Autodesk Fusion 360 part; units mm, degrees
(part 2 of 5)
sketch "草图10 (3)" plane through (0, 0, 26) normal (0, 0, 1) x (1, 0, 0) in component "L2_RemovableGrate"
  line L0 (329, 60.3) -> (333, 60.3)
  line L1 (333, 60.3) -> (333, 129.7)
  line L2 (333, 129.7) -> (329, 129.7)
  line L3 (329, 129.7) -> (329, 60.3)
  dimension "d585" = 329
  dimension "d587" = 4
  dimension "d588" = 69.4
  constraint horizontal L0
  constraint vertical L1
  constraint horizontal L2
  constraint vertical L3
  measures "d585" horizontal distance of origin L0.start
  measures "d587" horizontal distance of L0.start L0.end
  measures "d588" vertical distance of L0.end L1.end
extrude "Drain slot 9''" cut sketch "草图10 (3)" along normal blind 4 bodies 6 in component "L2_RemovableGrate"
ref_plane "工作平面11" through (0, 0, 26) normal (0, 0, 1) x (1, 0, 0) in component "L2_RemovableGrate"
sketch "草图11 (3)" plane through (0, 0, 26) normal (0, 0, 1) x (1, 0, 0) in component "L2_RemovableGrate"
  line L0 (339, 60.3) -> (343, 60.3)
  line L1 (343, 60.3) -> (343, 129.7)
  line L2 (343, 129.7) -> (339, 129.7)
  line L3 (339, 129.7) -> (339, 60.3)
  dimension "d593" = 339
  dimension "d595" = 4
  dimension "d596" = 69.4
  constraint horizontal L0
  constraint vertical L1
  constraint horizontal L2
  constraint vertical L3
  measures "d593" horizontal distance of origin L0.start
  measures "d595" horizontal distance of L0.start L0.end
  measures "d596" vertical distance of L0.end L1.end
extrude "Drain slot 10''" cut sketch "草图11 (3)" along normal blind 4 bodies 6 in component "L2_RemovableGrate"
ref_plane "工作平面12" through (0, 0, 26) normal (0, 0, 1) x (1, 0, 0) in component "L2_RemovableGrate"
sketch "草图12 (3)" plane through (0, 0, 26) normal (0, 0, 1) x (1, 0, 0) in component "L2_RemovableGrate"
  line L0 (349, 60.3) -> (353, 60.3)
  line L1 (353, 60.3) -> (353, 129.7)
  line L2 (353, 129.7) -> (349, 129.7)
  line L3 (349, 129.7) -> (349, 60.3)
  dimension "d601" = 349
  dimension "d603" = 4
  dimension "d604" = 69.4
  constraint horizontal L0
  constraint vertical L1
  constraint horizontal L2
  constraint vertical L3
  measures "d601" horizontal distance of origin L0.start
  measures "d603" horizontal distance of L0.start L0.end
  measures "d604" vertical distance of L0.end L1.end
extrude "Drain slot 11''" cut sketch "草图12 (3)" along normal blind 4 bodies 6 in component "L2_RemovableGrate"
ref_plane "工作平面13" through (0, 0, 26) normal (0, 0, 1) x (1, 0, 0) in component "L2_RemovableGrate"
sketch "草图13 (2)" plane through (0, 0, 26) normal (0, 0, 1) x (1, 0, 0) in component "L2_RemovableGrate"
  line L0 (359, 60.3) -> (363, 60.3)
  line L1 (363, 60.3) -> (363, 129.7)
  line L2 (363, 129.7) -> (359, 129.7)
  line L3 (359, 129.7) -> (359, 60.3)
  dimension "d609" = 359
  dimension "d611" = 4
  dimension "d612" = 69.4
  constraint horizontal L0
  constraint vertical L1
  constraint horizontal L2
  constraint vertical L3
  measures "d609" horizontal distance of origin L0.start
  measures "d611" horizontal distance of L0.start L0.end
  measures "d612" vertical distance of L0.end L1.end
extrude "Drain slot 12'" cut sketch "草图13 (2)" along normal blind 4 bodies 6 in component "L2_RemovableGrate"
ref_plane "工作平面14" through (0, 0, 26) normal (0, 0, 1) x (1, 0, 0) in component "L2_RemovableGrate"
sketch "草图14 (2)" plane through (0, 0, 26) normal (0, 0, 1) x (1, 0, 0) in component "L2_RemovableGrate"
  line L0 (369, 60.3) -> (373, 60.3)
  line L1 (373, 60.3) -> (373, 129.7)
  line L2 (373, 129.7) -> (369, 129.7)
  line L3 (369, 129.7) -> (369, 60.3)
  dimension "d617" = 369
  dimension "d619" = 4
  dimension "d620" = 69.4
  constraint horizontal L0
  constraint vertical L1
  constraint horizontal L2
  constraint vertical L3
  measures "d617" horizontal distance of origin L0.start
  measures "d619" horizontal distance of L0.start L0.end
  measures "d620" vertical distance of L0.end L1.end
extrude "Drain slot 13'" cut sketch "草图14 (2)" along normal blind 4 bodies 6 in component "L2_RemovableGrate"
ref_plane "工作平面15" through (0, 0, 26) normal (0, 0, 1) x (1, 0, 0) in component "L2_RemovableGrate"
sketch "草图15 (2)" plane through (0, 0, 26) normal (0, 0, 1) x (1, 0, 0) in component "L2_RemovableGrate"
  line L0 (379, 60.3) -> (383, 60.3)
  line L1 (383, 60.3) -> (383, 129.7)
  line L2 (383, 129.7) -> (379, 129.7)
  line L3 (379, 129.7) -> (379, 60.3)
  dimension "d625" = 379
  dimension "d627" = 4
  dimension "d628" = 69.4
  constraint horizontal L0
  constraint vertical L1
  constraint horizontal L2
  constraint vertical L3
  measures "d625" horizontal distance of origin L0.start
  measures "d627" horizontal distance of L0.start L0.end
  measures "d628" vertical distance of L0.end L1.end
extrude "Drain slot 14'" cut sketch "草图15 (2)" along normal blind 4 bodies 6 in component "L2_RemovableGrate"
ref_plane "工作平面16" through (0, 0, 26) normal (0, 0, 1) x (1, 0, 0) in component "L2_RemovableGrate"
sketch "草图16 (2)" plane through (0, 0, 26) normal (0, 0, 1) x (1, 0, 0) in component "L2_RemovableGrate"
  line L0 (389, 60.3) -> (393, 60.3)
  line L1 (393, 60.3) -> (393, 129.7)
  line L2 (393, 129.7) -> (389, 129.7)
  line L3 (389, 129.7) -> (389, 60.3)
  dimension "d633" = 389
  dimension "d635" = 4
  dimension "d636" = 69.4
  constraint horizontal L0
  constraint vertical L1
  constraint horizontal L2
  constraint vertical L3
  measures "d633" horizontal distance of origin L0.start
  measures "d635" horizontal distance of L0.start L0.end
  measures "d636" vertical distance of L0.end L1.end
extrude "Drain slot 15'" cut sketch "草图16 (2)" along normal blind 4 bodies 6 in component "L2_RemovableGrate"
ref_plane "工作平面17" through (0, 0, 26) normal (0, 0, 1) x (1, 0, 0) in component "L2_RemovableGrate"
sketch "草图17" plane through (0, 0, 26) normal (0, 0, 1) x (1, 0, 0) in component "L2_RemovableGrate"
  line L0 (399, 60.3) -> (403, 60.3)
  line L1 (403, 60.3) -> (403, 129.7)
  line L2 (403, 129.7) -> (399, 129.7)
  line L3 (399, 129.7) -> (399, 60.3)
  dimension "d641" = 399
  dimension "d643" = 4
  dimension "d644" = 69.4
  constraint horizontal L0
  constraint vertical L1
  constraint horizontal L2
  constraint vertical L3
  measures "d641" horizontal distance of origin L0.start
  measures "d643" horizontal distance of L0.start L0.end
  measures "d644" vertical distance of L0.end L1.end
extrude "Drain slot 16" cut sketch "草图17" along normal blind 4 bodies 6 in component "L2_RemovableGrate"
ref_plane "工作平面18" through (0, 0, 26) normal (0, 0, 1) x (1, 0, 0) in component "L2_RemovableGrate"
sketch "草图18" plane through (0, 0, 26) normal (0, 0, 1) x (1, 0, 0) in component "L2_RemovableGrate"
  line L0 (409, 60.3) -> (413, 60.3)
  line L1 (413, 60.3) -> (413, 129.7)
  line L2 (413, 129.7) -> (409, 129.7)
  line L3 (409, 129.7) -> (409, 60.3)
  dimension "d649" = 409
  dimension "d651" = 4
  dimension "d652" = 69.4
  constraint horizontal L0
  constraint vertical L1
  constraint horizontal L2
  constraint vertical L3
  measures "d649" horizontal distance of origin L0.start
  measures "d651" horizontal distance of L0.start L0.end
  measures "d652" vertical distance of L0.end L1.end
extrude "Drain slot 17" cut sketch "草图18" along normal blind 4 bodies 6 in component "L2_RemovableGrate"
chamfer "倒角1'''''" distance 0.4 angle 45 4 edges at (331, 136.7, 30) (426.7, 95, 30) (331, 53.3, 30) (235.3, 95, 30) on bodies 6 in component "L2_RemovableGrate"
ref_plane "工作平面1" through (0, 0, 10) normal (0, 0, 1) x (1, 0, 0) in component "R2_Integrated"
sketch "草图1 (7)" plane through (0, 0, 10) normal (0, 0, 1) x (1, 0, 0) in component "R2_Integrated"
  line L0 (726, 50) -> (860, 50)
  line L1 (860, 50) -> (860, 140)
  line L2 (860, 140) -> (726, 140)
  line L3 (726, 140) -> (726, 50)
  dimension "d658" = 726
  dimension "d659" = 50
  dimension "d660" = 134
  dimension "d661" = 90
  constraint horizontal L0
  constraint vertical L1
  constraint horizontal L2
  constraint vertical L3
  measures "d658" horizontal distance of origin L0.start
  measures "d659" vertical distance of origin L0.start
  measures "d660" horizontal distance of L0.start L0.end
  measures "d661" vertical distance of L0.end L1.end
extrude "R05 pan blank'''" add sketch "草图1 (7)" along normal blind 25 separate body makes body 7 in component "R2_Integrated"
fillet "Outside corner rounds'''" radius 3 4 edges at (726, 140, 22.5) (860, 140, 22.5) (860, 50, 22.5) (726, 50, 22.5) on bodies 7 in component "R2_Integrated"
ref_plane "工作平面2" through (729, 0, 0) normal (1, 0, 0) x (0, 1, 0) in component "R2_Integrated"
sketch "草图2 (7)" plane through (729, 0, 0) normal (1, 0, 0) x (0, 0, -1) in component "R2_Integrated"
  line L0 (-22.1441, 53) -> (-13, 140)
  line L1 (-13, 140) -> (-36, 140)
  line L2 (-36, 140) -> (-36, 53)
  line L3 (-36, 53) -> (-22.1441, 53)
  dimension "d670" = 13
  dimension "d672" = 36
  constraint horizontal L1
  constraint vertical L2
  constraint horizontal L3
  measures "d670" horizontal distance of origin L0.end
  measures "d672" horizontal distance of origin L1.end
extrude "R05 continuous slope and open edge'''" cut sketch "草图2 (7)" along normal blind 128 bodies 7 in component "R2_Integrated"
ref_plane "工作平面3" through (0, 0, 10) normal (0, 0, 1) x (1, 0, 0) in component "R2_Integrated"
sketch "草图3 (7)" plane through (0, 0, 10) normal (0, 0, 1) x (1, 0, 0) in component "R2_Integrated"
  line L0 (729, 53) -> (736, 65)
  line L1 (736, 65) -> (729, 77)
  line L2 (729, 77) -> (729, 53)
  dimension "d677" = 729
  dimension "d679" = 736
  dimension "d680" = 65
  constraint vertical L2
  measures "d677" horizontal distance of origin L0.start
  measures "d679" horizontal distance of origin L0.end
  measures "d680" vertical distance of origin L0.end
extrude "R05 triangular flow seat 00'''" add sketch "草图3 (7)" along normal blind 16 bodies 7 in component "R2_Integrated"
fillet "R05 soften flow seat tip'''" radius 1 1 edges at (736, 65, 23.4414) on bodies 7 in component "R2_Integrated"
ref_plane "工作平面4" through (0, 0, 10) normal (0, 0, 1) x (1, 0, 0) in component "R2_Integrated"
sketch "草图4 (7)" plane through (0, 0, 10) normal (0, 0, 1) x (1, 0, 0) in component "R2_Integrated"
  line L0 (729, 113) -> (736, 125)
  line L1 (736, 125) -> (729, 137)
  line L2 (729, 137) -> (729, 113)
  dimension "d688" = 729
  dimension "d690" = 736
  dimension "d691" = 125
  constraint vertical L2
  measures "d688" horizontal distance of origin L0.start
  measures "d690" horizontal distance of origin L0.end
  measures "d691" vertical distance of origin L0.end
extrude "R05 triangular flow seat 01'''" add sketch "草图4 (7)" along normal blind 16 bodies 7 in component "R2_Integrated"
fillet "R05 soften flow seat tip (1)'''" radius 1 1 edges at (736, 125, 20.2883) on bodies 7 in component "R2_Integrated"
ref_plane "工作平面5" through (0, 0, 10) normal (0, 0, 1) x (1, 0, 0) in component "R2_Integrated"
sketch "草图5 (7)" plane through (0, 0, 10) normal (0, 0, 1) x (1, 0, 0) in component "R2_Integrated"
  line L0 (857, 53) -> (850, 65)
  line L1 (850, 65) -> (857, 77)
  line L2 (857, 77) -> (857, 53)
  dimension "d699" = 857
  dimension "d701" = 850
  dimension "d702" = 65
  constraint vertical L2
  measures "d699" horizontal distance of origin L0.start
  measures "d701" horizontal distance of origin L0.end
  measures "d702" vertical distance of origin L0.end
extrude "R05 triangular flow seat 10'''" add sketch "草图5 (7)" along normal blind 16 bodies 7 in component "R2_Integrated"
fillet "R05 soften flow seat tip (2)'''" radius 1 1 edges at (850, 65, 23.4414) on bodies 7 in component "R2_Integrated"
ref_plane "工作平面6" through (0, 0, 10) normal (0, 0, 1) x (1, 0, 0) in component "R2_Integrated"
sketch "草图6 (7)" plane through (0, 0, 10) normal (0, 0, 1) x (1, 0, 0) in component "R2_Integrated"
  line L0 (857, 113) -> (850, 125)
  line L1 (850, 125) -> (857, 137)
  line L2 (857, 137) -> (857, 113)
  dimension "d710" = 857
  dimension "d712" = 850
  dimension "d713" = 125
  constraint vertical L2
  measures "d710" horizontal distance of origin L0.start
  measures "d712" horizontal distance of origin L0.end
  measures "d713" vertical distance of origin L0.end
extrude "R05 triangular flow seat 11'''" add sketch "草图6 (7)" along normal blind 16 bodies 7 in component "R2_Integrated"
fillet "R05 soften flow seat tip (3)'''" radius 1 1 edges at (850, 125, 20.2883) on bodies 7 in component "R2_Integrated"
ref_plane "工作平面7" through (0, 0, 0) normal (0, 0, 1) x (1, 0, 0) in component "R2_Integrated"
sketch "草图7 (7)" plane through (0, 0, 0) normal (0, 0, 1) x (1, 0, 0) in component "R2_Integrated"
  line L0 (729, 50) -> (737, 50)
  line L1 (737, 50) -> (737, 131)
  line L2 (737, 131) -> (729, 131)
  line L3 (729, 131) -> (729, 50)
  dimension "d721" = 729
  dimension "d722" = 50
  dimension "d723" = 8
  dimension "d724" = 81
  constraint horizontal L0
  constraint vertical L1
  constraint horizontal L2
  constraint vertical L3
  measures "d721" horizontal distance of origin L0.start
  measures "d722" vertical distance of origin L0.start
  measures "d723" horizontal distance of L0.start L0.end
  measures "d724" vertical distance of L0.end L1.end
extrude "R05 low integral runner 0'''" add sketch "草图7 (7)" along normal blind 10 bodies 7 in component "R2_Integrated"
ref_plane "工作平面8" through (0, 0, 0) normal (0, 0, 1) x (1, 0, 0) in component "R2_Integrated"
sketch "草图8 (7)" plane through (0, 0, 0) normal (0, 0, 1) x (1, 0, 0) in component "R2_Integrated"
  line L0 (849, 50) -> (857, 50)
  line L1 (857, 50) -> (857, 131)
  line L2 (857, 131) -> (849, 131)
  line L3 (849, 131) -> (849, 50)
  dimension "d729" = 849
  dimension "d730" = 50
  dimension "d731" = 8
  dimension "d732" = 81
  constraint horizontal L0
  constraint vertical L1
  constraint horizontal L2
  constraint vertical L3
  measures "d729" horizontal distance of origin L0.start
  measures "d730" vertical distance of origin L0.start
  measures "d731" horizontal distance of L0.start L0.end
  measures "d732" vertical distance of L0.end L1.end
extrude "R05 low integral runner 1'''" add sketch "草图8 (7)" along normal blind 10 bodies 7 in component "R2_Integrated"
chamfer "倒角1''''''" distance 0.4 angle 45 5 edges at (729, 96.5, 35) (857, 96.5, 35) (793, 53, 35) (726, 95, 35) (860, 95, 35) on bodies 7 in component "R2_Integrated"
ref_plane "工作平面1" through (0, 0, 26) normal (0, 0, 1) x (1, 0, 0) in component "R2_RemovableGrate"
sketch "草图1 (8)" plane through (0, 0, 26) normal (0, 0, 1) x (1, 0, 0) in component "R2_RemovableGrate"
  line L0 (729.3, 53.3) -> (856.7, 53.3)
  line L1 (856.7, 53.3) -> (856.7, 136.7)
  line L2 (856.7, 136.7) -> (729.3, 136.7)
  line L3 (729.3, 136.7) -> (729.3, 53.3)
  dimension "d738" = 729.3
  dimension "d740" = 127.4
  dimension "d741" = 83.4
  constraint horizontal L0
  constraint vertical L1
  constraint horizontal L2
  constraint vertical L3
  measures "d738" horizontal distance of origin L0.start
  measures "d740" horizontal distance of L0.start L0.end
  measures "d741" vertical distance of L0.end L1.end
extrude "Horizontal removable deck'''" add sketch "草图1 (8)" along normal blind 4 separate body makes body 8 in component "R2_RemovableGrate"
ref_plane "工作平面2" through (0, 0, 26) normal (0, 0, 1) x (1, 0, 0) in component "R2_RemovableGrate"
sketch "草图2 (8)" plane through (0, 0, 26) normal (0, 0, 1) x (1, 0, 0) in component "R2_RemovableGrate"
  line L0 (741, 60.3) -> (745, 60.3)
  line L1 (745, 60.3) -> (745, 129.7)
  line L2 (745, 129.7) -> (741, 129.7)
  line L3 (741, 129.7) -> (741, 60.3)
  dimension "d746" = 741
  dimension "d748" = 4
  dimension "d749" = 69.4
  constraint horizontal L0
  constraint vertical L1
  constraint horizontal L2
  constraint vertical L3
  measures "d746" horizontal distance of origin L0.start
  measures "d748" horizontal distance of L0.start L0.end
  measures "d749" vertical distance of L0.end L1.end
extrude "Drain slot 1'''" cut sketch "草图2 (8)" along normal blind 4 bodies 8 in component "R2_RemovableGrate"
ref_plane "工作平面3" through (0, 0, 26) normal (0, 0, 1) x (1, 0, 0) in component "R2_RemovableGrate"
sketch "草图3 (8)" plane through (0, 0, 26) normal (0, 0, 1) x (1, 0, 0) in component "R2_RemovableGrate"
  line L0 (751, 60.3) -> (755, 60.3)
  line L1 (755, 60.3) -> (755, 129.7)
  line L2 (755, 129.7) -> (751, 129.7)
  line L3 (751, 129.7) -> (751, 60.3)
  dimension "d754" = 751
  dimension "d756" = 4
  dimension "d757" = 69.4
  constraint horizontal L0
  constraint vertical L1
  constraint horizontal L2
  constraint vertical L3
  measures "d754" horizontal distance of origin L0.start
  measures "d756" horizontal distance of L0.start L0.end
  measures "d757" vertical distance of L0.end L1.end
extrude "Drain slot 2'''" cut sketch "草图3 (8)" along normal blind 4 bodies 8 in component "R2_RemovableGrate"
ref_plane "工作平面4" through (0, 0, 26) normal (0, 0, 1) x (1, 0, 0) in component "R2_RemovableGrate"
sketch "草图4 (8)" plane through (0, 0, 26) normal (0, 0, 1) x (1, 0, 0) in component "R2_RemovableGrate"
  line L0 (761, 60.3) -> (765, 60.3)
  line L1 (765, 60.3) -> (765, 129.7)
  line L2 (765, 129.7) -> (761, 129.7)
  line L3 (761, 129.7) -> (761, 60.3)
  dimension "d762" = 761
  dimension "d764" = 4
  dimension "d765" = 69.4
  constraint horizontal L0
  constraint vertical L1
  constraint horizontal L2
  constraint vertical L3
  measures "d762" horizontal distance of origin L0.start
  measures "d764" horizontal distance of L0.start L0.end
  measures "d765" vertical distance of L0.end L1.end
extrude "Drain slot 3'''" cut sketch "草图4 (8)" along normal blind 4 bodies 8 in component "R2_RemovableGrate"
ref_plane "工作平面5" through (0, 0, 26) normal (0, 0, 1) x (1, 0, 0) in component "R2_RemovableGrate"
sketch "草图5 (8)" plane through (0, 0, 26) normal (0, 0, 1) x (1, 0, 0) in component "R2_RemovableGrate"
  line L0 (771, 60.3) -> (775, 60.3)
  line L1 (775, 60.3) -> (775, 129.7)
  line L2 (775, 129.7) -> (771, 129.7)
  line L3 (771, 129.7) -> (771, 60.3)
  dimension "d770" = 771
  dimension "d772" = 4
  dimension "d773" = 69.4
  constraint horizontal L0
  constraint vertical L1
  constraint horizontal L2
  constraint vertical L3
  measures "d770" horizontal distance of origin L0.start
  measures "d772" horizontal distance of L0.start L0.end
  measures "d773" vertical distance of L0.end L1.end
extrude "Drain slot 4'''" cut sketch "草图5 (8)" along normal blind 4 bodies 8 in component "R2_RemovableGrate"
ref_plane "工作平面6" through (0, 0, 26) normal (0, 0, 1) x (1, 0, 0) in component "R2_RemovableGrate"
sketch "草图6 (8)" plane through (0, 0, 26) normal (0, 0, 1) x (1, 0, 0) in component "R2_RemovableGrate"
  line L0 (781, 60.3) -> (785, 60.3)
  line L1 (785, 60.3) -> (785, 129.7)
  line L2 (785, 129.7) -> (781, 129.7)
  line L3 (781, 129.7) -> (781, 60.3)
  dimension "d778" = 781
  dimension "d780" = 4
  dimension "d781" = 69.4
  constraint horizontal L0
  constraint vertical L1
  constraint horizontal L2
  constraint vertical L3
  measures "d778" horizontal distance of origin L0.start
  measures "d780" horizontal distance of L0.start L0.end
  measures "d781" vertical distance of L0.end L1.end
extrude "Drain slot 5'''" cut sketch "草图6 (8)" along normal blind 4 bodies 8 in component "R2_RemovableGrate"
ref_plane "工作平面7" through (0, 0, 26) normal (0, 0, 1) x (1, 0, 0) in component "R2_RemovableGrate"
sketch "草图7 (8)" plane through (0, 0, 26) normal (0, 0, 1) x (1, 0, 0) in component "R2_RemovableGrate"
  line L0 (791, 60.3) -> (795, 60.3)
  line L1 (795, 60.3) -> (795, 129.7)
  line L2 (795, 129.7) -> (791, 129.7)
  line L3 (791, 129.7) -> (791, 60.3)
  dimension "d786" = 791
  dimension "d788" = 4
  dimension "d789" = 69.4
  constraint horizontal L0
  constraint vertical L1
  constraint horizontal L2
  constraint vertical L3
  measures "d786" horizontal distance of origin L0.start
  measures "d788" horizontal distance of L0.start L0.end
  measures "d789" vertical distance of L0.end L1.end
extrude "Drain slot 6'''" cut sketch "草图7 (8)" along normal blind 4 bodies 8 in component "R2_RemovableGrate"
ref_plane "工作平面8" through (0, 0, 26) normal (0, 0, 1) x (1, 0, 0) in component "R2_RemovableGrate"
sketch "草图8 (8)" plane through (0, 0, 26) normal (0, 0, 1) x (1, 0, 0) in component "R2_RemovableGrate"
  line L0 (801, 60.3) -> (805, 60.3)
  line L1 (805, 60.3) -> (805, 129.7)
  line L2 (805, 129.7) -> (801, 129.7)
  line L3 (801, 129.7) -> (801, 60.3)
  dimension "d794" = 801
  dimension "d796" = 4
  dimension "d797" = 69.4
  constraint horizontal L0
  constraint vertical L1
  constraint horizontal L2
  constraint vertical L3
  measures "d794" horizontal distance of origin L0.start
  measures "d796" horizontal distance of L0.start L0.end
  measures "d797" vertical distance of L0.end L1.end
extrude "Drain slot 7'''" cut sketch "草图8 (8)" along normal blind 4 bodies 8 in component "R2_RemovableGrate"
ref_plane "工作平面9" through (0, 0, 26) normal (0, 0, 1) x (1, 0, 0) in component "R2_RemovableGrate"
sketch "草图9 (4)" plane through (0, 0, 26) normal (0, 0, 1) x (1, 0, 0) in component "R2_RemovableGrate"
  line L0 (811, 60.3) -> (815, 60.3)
  line L1 (815, 60.3) -> (815, 129.7)
  line L2 (815, 129.7) -> (811, 129.7)
  line L3 (811, 129.7) -> (811, 60.3)
  dimension "d802" = 811
  dimension "d804" = 4
  dimension "d805" = 69.4
  constraint horizontal L0
  constraint vertical L1
  constraint horizontal L2
  constraint vertical L3
  measures "d802" horizontal distance of origin L0.start
  measures "d804" horizontal distance of L0.start L0.end
  measures "d805" vertical distance of L0.end L1.end
extrude "Drain slot 8'''" cut sketch "草图9 (4)" along normal blind 4 bodies 8 in component "R2_RemovableGrate"
ref_plane "工作平面10" through (0, 0, 26) normal (0, 0, 1) x (1, 0, 0) in component "R2_RemovableGrate"
sketch "草图10 (4)" plane through (0, 0, 26) normal (0, 0, 1) x (1, 0, 0) in component "R2_RemovableGrate"
  line L0 (821, 60.3) -> (825, 60.3)
  line L1 (825, 60.3) -> (825, 129.7)
  line L2 (825, 129.7) -> (821, 129.7)
  line L3 (821, 129.7) -> (821, 60.3)
  dimension "d810" = 821
  dimension "d812" = 4
  dimension "d813" = 69.4
  constraint horizontal L0
  constraint vertical L1
  constraint horizontal L2
  constraint vertical L3
  measures "d810" horizontal distance of origin L0.start
  measures "d812" horizontal distance of L0.start L0.end
  measures "d813" vertical distance of L0.end L1.end
extrude "Drain slot 9'''" cut sketch "草图10 (4)" along normal blind 4 bodies 8 in component "R2_RemovableGrate"
ref_plane "工作平面11" through (0, 0, 26) normal (0, 0, 1) x (1, 0, 0) in component "R2_RemovableGrate"
sketch "草图11 (4)" plane through (0, 0, 26) normal (0, 0, 1) x (1, 0, 0) in component "R2_RemovableGrate"
  line L0 (831, 60.3) -> (835, 60.3)
  line L1 (835, 60.3) -> (835, 129.7)
  line L2 (835, 129.7) -> (831, 129.7)
  line L3 (831, 129.7) -> (831, 60.3)
  dimension "d818" = 831
  dimension "d820" = 4
  dimension "d821" = 69.4
  constraint horizontal L0
  constraint vertical L1
  constraint horizontal L2
  constraint vertical L3
  measures "d818" horizontal distance of origin L0.start
  measures "d820" horizontal distance of L0.start L0.end
  measures "d821" vertical distance of L0.end L1.end
extrude "Drain slot 10'''" cut sketch "草图11 (4)" along normal blind 4 bodies 8 in component "R2_RemovableGrate"
ref_plane "工作平面12" through (0, 0, 26) normal (0, 0, 1) x (1, 0, 0) in component "R2_RemovableGrate"
sketch "草图12 (4)" plane through (0, 0, 26) normal (0, 0, 1) x (1, 0, 0) in component "R2_RemovableGrate"
  line L0 (841, 60.3) -> (845, 60.3)
  line L1 (845, 60.3) -> (845, 129.7)
  line L2 (845, 129.7) -> (841, 129.7)
  line L3 (841, 129.7) -> (841, 60.3)
  dimension "d826" = 841
  dimension "d828" = 4
  dimension "d829" = 69.4
  constraint horizontal L0
  constraint vertical L1
  constraint horizontal L2
  constraint vertical L3
  measures "d826" horizontal distance of origin L0.start
  measures "d828" horizontal distance of L0.start L0.end
  measures "d829" vertical distance of L0.end L1.end
extrude "Drain slot 11'''" cut sketch "草图12 (4)" along normal blind 4 bodies 8 in component "R2_RemovableGrate"
chamfer "倒角1'''''''" distance 0.4 angle 45 4 edges at (793, 136.7, 30) (856.7, 95, 30) (793, 53.3, 30) (729.3, 95, 30) on bodies 8 in component "R2_RemovableGrate"
ref_plane "工作平面1" through (0, 0, 10) normal (0, 0, 1) x (1, 0, 0) in component "LS_Integrated"
sketch "草图1 (9)" plane through (0, 0, 10) normal (0, 0, 1) x (1, 0, 0) in component "LS_Integrated"
  line L0 (50, 142) -> (170, 142)
  line L1 (170, 142) -> (170, 322)
  line L2 (170, 322) -> (50, 322)
  line L3 (50, 322) -> (50, 142)
  dimension "d835" = 50
  dimension "d836" = 142
  dimension "d837" = 120
  dimension "d838" = 180
  constraint horizontal L0
  constraint vertical L1
  constraint horizontal L2
  constraint vertical L3
  measures "d835" horizontal distance of origin L0.start
  measures "d836" vertical distance of origin L0.start
  measures "d837" horizontal distance of L0.start L0.end
  measures "d838" vertical distance of L0.end L1.end
extrude "R05 pan blank''''" add sketch "草图1 (9)" along normal blind 25 separate body makes body 9 in component "LS_Integrated"
fillet "Outside corner rounds''''" radius 3 4 edges at (50, 322, 22.5) (170, 322, 22.5) (170, 142, 22.5) (50, 142, 22.5) on bodies 9 in component "LS_Integrated"
ref_plane "工作平面2" through (0, 319, 0) normal (0, 1, 0) x (0, 0, 1) in component "LS_Integrated"
sketch "草图2 (9)" plane through (0, 319, 0) normal (0, 1, 0) x (1, 0, 0) in component "LS_Integrated"
  line L0 (53, -25.2972) -> (170, -13)
  line L1 (170, -13) -> (170, -36)
  line L2 (170, -36) -> (53, -36)
  line L3 (53, -36) -> (53, -25.2972)
  dimension "d846" = 25.2972
  dimension "d848" = 13
  dimension "d849" = 36
  constraint vertical L1
  constraint horizontal L2
  constraint vertical L3
  measures "d846" vertical distance of origin L0.start
  measures "d848" vertical distance of origin L0.end
  measures "d849" vertical distance of origin L1.end
extrude "R05 continuous slope and open edge''''" cut sketch "草图2 (9)" against normal blind 174 bodies 9 in component "LS_Integrated"
ref_plane "工作平面3" through (0, 0, 10) normal (0, 0, 1) x (1, 0, 0) in component "LS_Integrated"
sketch "草图3 (9)" plane through (0, 0, 10) normal (0, 0, 1) x (1, 0, 0) in component "LS_Integrated"
  line L0 (53, 319) -> (65, 312)
  line L1 (65, 312) -> (77, 319)
  line L2 (77, 319) -> (53, 319)
  dimension "d856" = 65
  constraint horizontal L2
  measures "d856" horizontal distance of origin L0.end
extrude "R05 triangular flow seat 00''''" add sketch "草图3 (9)" along normal blind 16 bodies 9 in component "LS_Integrated"
fillet "R05 soften flow seat tip''''" radius 1 1 edges at (65, 312, 25.018) on bodies 9 in component "LS_Integrated"
ref_plane "工作平面4" through (0, 0, 10) normal (0, 0, 1) x (1, 0, 0) in component "LS_Integrated"
sketch "草图4 (9)" plane through (0, 0, 10) normal (0, 0, 1) x (1, 0, 0) in component "LS_Integrated"
  line L0 (143, 319) -> (155, 312)
  line L1 (155, 312) -> (167, 319)
  line L2 (167, 319) -> (143, 319)
  dimension "d867" = 155
  constraint horizontal L2
  measures "d867" horizontal distance of origin L0.end
extrude "R05 triangular flow seat 01''''" add sketch "草图4 (9)" along normal blind 16 bodies 9 in component "LS_Integrated"
fillet "R05 soften flow seat tip (1)''''" radius 1 1 edges at (155, 312, 20.2883) on bodies 9 in component "LS_Integrated"
ref_plane "工作平面5" through (0, 0, 10) normal (0, 0, 1) x (1, 0, 0) in component "LS_Integrated"
sketch "草图5 (9)" plane through (0, 0, 10) normal (0, 0, 1) x (1, 0, 0) in component "LS_Integrated"
  line L0 (53, 145) -> (65, 152)
  line L1 (65, 152) -> (77, 145)
  line L2 (77, 145) -> (53, 145)
  dimension "d878" = 65
  dimension "d879" = 152
  constraint horizontal L2
  measures "d878" horizontal distance of origin L0.end
  measures "d879" vertical distance of origin L0.end
extrude "R05 triangular flow seat 10''''" add sketch "草图5 (9)" along normal blind 16 bodies 9 in component "LS_Integrated"
fillet "R05 soften flow seat tip (2)''''" radius 1 1 edges at (65, 152, 25.018) on bodies 9 in component "LS_Integrated"
ref_plane "工作平面6" through (0, 0, 10) normal (0, 0, 1) x (1, 0, 0) in component "LS_Integrated"
sketch "草图6 (9)" plane through (0, 0, 10) normal (0, 0, 1) x (1, 0, 0) in component "LS_Integrated"
  line L0 (143, 145) -> (155, 152)
  line L1 (155, 152) -> (167, 145)
  line L2 (167, 145) -> (143, 145)
  dimension "d889" = 155
  dimension "d890" = 152
  constraint horizontal L2
  measures "d889" horizontal distance of origin L0.end
  measures "d890" vertical distance of origin L0.end
extrude "R05 triangular flow seat 11''''" add sketch "草图6 (9)" along normal blind 16 bodies 9 in component "LS_Integrated"
fillet "R05 soften flow seat tip (3)''''" radius 1 1 edges at (155, 152, 20.2883) on bodies 9 in component "LS_Integrated"
ref_plane "工作平面7" through (0, 0, 0) normal (0, 0, 1) x (1, 0, 0) in component "LS_Integrated"
sketch "草图7 (9)" plane through (0, 0, 0) normal (0, 0, 1) x (1, 0, 0) in component "LS_Integrated"
  line L0 (50, 311) -> (161, 311)
  line L1 (161, 311) -> (161, 319)
  line L2 (161, 319) -> (50, 319)
  line L3 (50, 319) -> (50, 311)
  dimension "d898" = 50
  dimension "d899" = 311
  dimension "d900" = 111
  dimension "d901" = 8
  constraint horizontal L0
  constraint vertical L1
  constraint horizontal L2
  constraint vertical L3
  measures "d898" horizontal distance of origin L0.start
  measures "d899" vertical distance of origin L0.start
  measures "d900" horizontal distance of L0.start L0.end
  measures "d901" vertical distance of L0.end L1.end
extrude "R05 low integral runner 0''''" add sketch "草图7 (9)" along normal blind 10 bodies 9 in component "LS_Integrated"
ref_plane "工作平面8" through (0, 0, 0) normal (0, 0, 1) x (1, 0, 0) in component "LS_Integrated"
sketch "草图8 (9)" plane through (0, 0, 0) normal (0, 0, 1) x (1, 0, 0) in component "LS_Integrated"
  line L0 (50, 145) -> (161, 145)
  line L1 (161, 145) -> (161, 153)
  line L2 (161, 153) -> (50, 153)
  line L3 (50, 153) -> (50, 145)
  dimension "d906" = 50
  dimension "d907" = 145
  dimension "d908" = 111
  dimension "d909" = 8
  constraint horizontal L0
  constraint vertical L1
  constraint horizontal L2
  constraint vertical L3
  measures "d906" horizontal distance of origin L0.start
  measures "d907" vertical distance of origin L0.start
  measures "d908" horizontal distance of L0.start L0.end
  measures "d909" vertical distance of L0.end L1.end
extrude "R05 low integral runner 1''''" add sketch "草图8 (9)" along normal blind 10 bodies 9 in component "LS_Integrated"
chamfer "倒角1''''''''" distance 0.4 angle 45 5 edges at (111.5, 319, 35) (111.5, 145, 35) (53, 232, 35) (110, 322, 35) (110, 142, 35) on bodies 9 in component "LS_Integrated"
ref_plane "工作平面1" through (0, 0, 26) normal (0, 0, 1) x (1, 0, 0) in component "LS_RemovableGrate"
sketch "草图1 (10)" plane through (0, 0, 26) normal (0, 0, 1) x (1, 0, 0) in component "LS_RemovableGrate"
  line L0 (53.3, 145.3) -> (166.7, 145.3)
  line L1 (166.7, 145.3) -> (166.7, 318.7)
  line L2 (166.7, 318.7) -> (53.3, 318.7)
  line L3 (53.3, 318.7) -> (53.3, 145.3)
  dimension "d916" = 145.3
  dimension "d917" = 113.4
  dimension "d918" = 173.4
  constraint horizontal L0
  constraint vertical L1
  constraint horizontal L2
  constraint vertical L3
  measures "d916" vertical distance of origin L0.start
  measures "d917" horizontal distance of L0.start L0.end
  measures "d918" vertical distance of L0.end L1.end
extrude "Horizontal removable deck''''" add sketch "草图1 (10)" along normal blind 4 separate body makes body 10 in component "LS_RemovableGrate"
ref_plane "工作平面2" through (0, 0, 26) normal (0, 0, 1) x (1, 0, 0) in component "LS_RemovableGrate"
sketch "草图2 (10)" plane through (0, 0, 26) normal (0, 0, 1) x (1, 0, 0) in component "LS_RemovableGrate"
  line L0 (60.3, 300) -> (159.7, 300)
  line L1 (159.7, 300) -> (159.7, 304)
  line L2 (159.7, 304) -> (60.3, 304)
  line L3 (60.3, 304) -> (60.3, 300)
  dimension "d924" = 300
  dimension "d925" = 99.4
  dimension "d926" = 4
  constraint horizontal L0
  constraint vertical L1
  constraint horizontal L2
  constraint vertical L3
  measures "d924" vertical distance of origin L0.start
  measures "d925" horizontal distance of L0.start L0.end
  measures "d926" vertical distance of L0.end L1.end
extrude "Drain slot 1''''" cut sketch "草图2 (10)" along normal blind 4 bodies 10 in component "LS_RemovableGrate"
ref_plane "工作平面3" through (0, 0, 26) normal (0, 0, 1) x (1, 0, 0) in component "LS_RemovableGrate"
sketch "草图3 (10)" plane through (0, 0, 26) normal (0, 0, 1) x (1, 0, 0) in component "LS_RemovableGrate"
  line L0 (60.3, 290) -> (159.7, 290)
  line L1 (159.7, 290) -> (159.7, 294)
  line L2 (159.7, 294) -> (60.3, 294)
  line L3 (60.3, 294) -> (60.3, 290)
  dimension "d932" = 290
  dimension "d933" = 99.4
  dimension "d934" = 4
  constraint horizontal L0
  constraint vertical L1
  constraint horizontal L2
  constraint vertical L3
  measures "d932" vertical distance of origin L0.start
  measures "d933" horizontal distance of L0.start L0.end
  measures "d934" vertical distance of L0.end L1.end
extrude "Drain slot 2''''" cut sketch "草图3 (10)" along normal blind 4 bodies 10 in component "LS_RemovableGrate"
ref_plane "工作平面4" through (0, 0, 26) normal (0, 0, 1) x (1, 0, 0) in component "LS_RemovableGrate"
sketch "草图4 (10)" plane through (0, 0, 26) normal (0, 0, 1) x (1, 0, 0) in component "LS_RemovableGrate"
  line L0 (60.3, 280) -> (159.7, 280)
  line L1 (159.7, 280) -> (159.7, 284)
  line L2 (159.7, 284) -> (60.3, 284)
  line L3 (60.3, 284) -> (60.3, 280)
  dimension "d940" = 280
  dimension "d941" = 99.4
  dimension "d942" = 4
  constraint horizontal L0
  constraint vertical L1
  constraint horizontal L2
  constraint vertical L3
  measures "d940" vertical distance of origin L0.start
  measures "d941" horizontal distance of L0.start L0.end
  measures "d942" vertical distance of L0.end L1.end
extrude "Drain slot 3''''" cut sketch "草图4 (10)" along normal blind 4 bodies 10 in component "LS_RemovableGrate"
ref_plane "工作平面5" through (0, 0, 26) normal (0, 0, 1) x (1, 0, 0) in component "LS_RemovableGrate"
sketch "草图5 (10)" plane through (0, 0, 26) normal (0, 0, 1) x (1, 0, 0) in component "LS_RemovableGrate"
  line L0 (60.3, 270) -> (159.7, 270)
  line L1 (159.7, 270) -> (159.7, 274)
  line L2 (159.7, 274) -> (60.3, 274)
  line L3 (60.3, 274) -> (60.3, 270)
  dimension "d948" = 270
  dimension "d949" = 99.4
  dimension "d950" = 4
  constraint horizontal L0
  constraint vertical L1
  constraint horizontal L2
  constraint vertical L3
  measures "d948" vertical distance of origin L0.start
  measures "d949" horizontal distance of L0.start L0.end
  measures "d950" vertical distance of L0.end L1.end
extrude "Drain slot 4''''" cut sketch "草图5 (10)" along normal blind 4 bodies 10 in component "LS_RemovableGrate"
ref_plane "工作平面6" through (0, 0, 26) normal (0, 0, 1) x (1, 0, 0) in component "LS_RemovableGrate"
sketch "草图6 (10)" plane through (0, 0, 26) normal (0, 0, 1) x (1, 0, 0) in component "LS_RemovableGrate"
  line L0 (60.3, 260) -> (159.7, 260)
  line L1 (159.7, 260) -> (159.7, 264)
  line L2 (159.7, 264) -> (60.3, 264)
  line L3 (60.3, 264) -> (60.3, 260)
  dimension "d956" = 260
  dimension "d957" = 99.4
  dimension "d958" = 4
  constraint horizontal L0
  constraint vertical L1
  constraint horizontal L2
  constraint vertical L3
  measures "d956" vertical distance of origin L0.start
  measures "d957" horizontal distance of L0.start L0.end
  measures "d958" vertical distance of L0.end L1.end
extrude "Drain slot 5''''" cut sketch "草图6 (10)" along normal blind 4 bodies 10 in component "LS_RemovableGrate"
ref_plane "工作平面7" through (0, 0, 26) normal (0, 0, 1) x (1, 0, 0) in component "LS_RemovableGrate"
sketch "草图7 (10)" plane through (0, 0, 26) normal (0, 0, 1) x (1, 0, 0) in component "LS_RemovableGrate"
  line L0 (60.3, 250) -> (159.7, 250)
  line L1 (159.7, 250) -> (159.7, 254)
  line L2 (159.7, 254) -> (60.3, 254)
  line L3 (60.3, 254) -> (60.3, 250)
  dimension "d964" = 250
  dimension "d965" = 99.4
  dimension "d966" = 4
  constraint horizontal L0
  constraint vertical L1
  constraint horizontal L2
  constraint vertical L3
  measures "d964" vertical distance of origin L0.start
  measures "d965" horizontal distance of L0.start L0.end
  measures "d966" vertical distance of L0.end L1.end
extrude "Drain slot 6''''" cut sketch "草图7 (10)" along normal blind 4 bodies 10 in component "LS_RemovableGrate"
ref_plane "工作平面8" through (0, 0, 26) normal (0, 0, 1) x (1, 0, 0) in component "LS_RemovableGrate"
sketch "草图8 (10)" plane through (0, 0, 26) normal (0, 0, 1) x (1, 0, 0) in component "LS_RemovableGrate"
  line L0 (60.3, 240) -> (159.7, 240)
  line L1 (159.7, 240) -> (159.7, 244)
  line L2 (159.7, 244) -> (60.3, 244)
  line L3 (60.3, 244) -> (60.3, 240)
  dimension "d972" = 240
  dimension "d973" = 99.4
  dimension "d974" = 4
  constraint horizontal L0
  constraint vertical L1
  constraint horizontal L2
  constraint vertical L3
  measures "d972" vertical distance of origin L0.start
  measures "d973" horizontal distance of L0.start L0.end
  measures "d974" vertical distance of L0.end L1.end
extrude "Drain slot 7''''" cut sketch "草图8 (10)" along normal blind 4 bodies 10 in component "LS_RemovableGrate"
ref_plane "工作平面9" through (0, 0, 26) normal (0, 0, 1) x (1, 0, 0) in component "LS_RemovableGrate"
sketch "草图9 (5)" plane through (0, 0, 26) normal (0, 0, 1) x (1, 0, 0) in component "LS_RemovableGrate"
  line L0 (60.3, 230) -> (159.7, 230)
  line L1 (159.7, 230) -> (159.7, 234)
  line L2 (159.7, 234) -> (60.3, 234)
  line L3 (60.3, 234) -> (60.3, 230)
  dimension "d980" = 230
  dimension "d981" = 99.4
  dimension "d982" = 4
  constraint horizontal L0
  constraint vertical L1
  constraint horizontal L2
  constraint vertical L3
  measures "d980" vertical distance of origin L0.start
  measures "d981" horizontal distance of L0.start L0.end
  measures "d982" vertical distance of L0.end L1.end
extrude "Drain slot 8''''" cut sketch "草图9 (5)" along normal blind 4 bodies 10 in component "LS_RemovableGrate"
ref_plane "工作平面10" through (0, 0, 26) normal (0, 0, 1) x (1, 0, 0) in component "LS_RemovableGrate"
sketch "草图10 (5)" plane through (0, 0, 26) normal (0, 0, 1) x (1, 0, 0) in component "LS_RemovableGrate"
  line L0 (60.3, 220) -> (159.7, 220)
  line L1 (159.7, 220) -> (159.7, 224)
  line L2 (159.7, 224) -> (60.3, 224)
  line L3 (60.3, 224) -> (60.3, 220)
  dimension "d988" = 220
  dimension "d989" = 99.4
  dimension "d990" = 4
  constraint horizontal L0
  constraint vertical L1
  constraint horizontal L2
  constraint vertical L3
  measures "d988" vertical distance of origin L0.start
  measures "d989" horizontal distance of L0.start L0.end
  measures "d990" vertical distance of L0.end L1.end
extrude "Drain slot 9''''" cut sketch "草图10 (5)" along normal blind 4 bodies 10 in component "LS_RemovableGrate"
ref_plane "工作平面11" through (0, 0, 26) normal (0, 0, 1) x (1, 0, 0) in component "LS_RemovableGrate"
sketch "草图11 (5)" plane through (0, 0, 26) normal (0, 0, 1) x (1, 0, 0) in component "LS_RemovableGrate"
  line L0 (60.3, 210) -> (159.7, 210)
  line L1 (159.7, 210) -> (159.7, 214)
  line L2 (159.7, 214) -> (60.3, 214)
  line L3 (60.3, 214) -> (60.3, 210)
  dimension "d996" = 210
  dimension "d997" = 99.4
  dimension "d998" = 4
  constraint horizontal L0
  constraint vertical L1
  constraint horizontal L2
  constraint vertical L3
  measures "d996" vertical distance of origin L0.start
  measures "d997" horizontal distance of L0.start L0.end
  measures "d998" vertical distance of L0.end L1.end
extrude "Drain slot 10''''" cut sketch "草图11 (5)" along normal blind 4 bodies 10 in component "LS_RemovableGrate"
ref_plane "工作平面12" through (0, 0, 26) normal (0, 0, 1) x (1, 0, 0) in component "LS_RemovableGrate"
sketch "草图12 (5)" plane through (0, 0, 26) normal (0, 0, 1) x (1, 0, 0) in component "LS_RemovableGrate"
  line L0 (60.3, 200) -> (159.7, 200)
  line L1 (159.7, 200) -> (159.7, 204)
  line L2 (159.7, 204) -> (60.3, 204)
  line L3 (60.3, 204) -> (60.3, 200)
  dimension "d1004" = 200
  dimension "d1005" = 99.4
  dimension "d1006" = 4
  constraint horizontal L0
  constraint vertical L1
  constraint horizontal L2
  constraint vertical L3
  measures "d1004" vertical distance of origin L0.start
  measures "d1005" horizontal distance of L0.start L0.end
  measures "d1006" vertical distance of L0.end L1.end
extrude "Drain slot 11''''" cut sketch "草图12 (5)" along normal blind 4 bodies 10 in component "LS_RemovableGrate"
ref_plane "工作平面13" through (0, 0, 26) normal (0, 0, 1) x (1, 0, 0) in component "LS_RemovableGrate"
sketch "草图13 (3)" plane through (0, 0, 26) normal (0, 0, 1) x (1, 0, 0) in component "LS_RemovableGrate"
  line L0 (60.3, 190) -> (159.7, 190)
  line L1 (159.7, 190) -> (159.7, 194)
  line L2 (159.7, 194) -> (60.3, 194)
  line L3 (60.3, 194) -> (60.3, 190)
  dimension "d1012" = 190
  dimension "d1013" = 99.4
  dimension "d1014" = 4
  constraint horizontal L0
  constraint vertical L1
  constraint horizontal L2
  constraint vertical L3
  measures "d1012" vertical distance of origin L0.start
  measures "d1013" horizontal distance of L0.start L0.end
  measures "d1014" vertical distance of L0.end L1.end
extrude "Drain slot 12''" cut sketch "草图13 (3)" along normal blind 4 bodies 10 in component "LS_RemovableGrate"
ref_plane "工作平面14" through (0, 0, 26) normal (0, 0, 1) x (1, 0, 0) in component "LS_RemovableGrate"
sketch "草图14 (3)" plane through (0, 0, 26) normal (0, 0, 1) x (1, 0, 0) in component "LS_RemovableGrate"
  line L0 (60.3, 180) -> (159.7, 180)
  line L1 (159.7, 180) -> (159.7, 184)
  line L2 (159.7, 184) -> (60.3, 184)
  line L3 (60.3, 184) -> (60.3, 180)
  dimension "d1020" = 180
  dimension "d1021" = 99.4
  dimension "d1022" = 4
  constraint horizontal L0
  constraint vertical L1
  constraint horizontal L2
  constraint vertical L3
  measures "d1020" vertical distance of origin L0.start
  measures "d1021" horizontal distance of L0.start L0.end
  measures "d1022" vertical distance of L0.end L1.end
extrude "Drain slot 13''" cut sketch "草图14 (3)" along normal blind 4 bodies 10 in component "LS_RemovableGrate"
ref_plane "工作平面15" through (0, 0, 26) normal (0, 0, 1) x (1, 0, 0) in component "LS_RemovableGrate"
sketch "草图15 (3)" plane through (0, 0, 26) normal (0, 0, 1) x (1, 0, 0) in component "LS_RemovableGrate"
  line L0 (60.3, 170) -> (159.7, 170)
  line L1 (159.7, 170) -> (159.7, 174)
  line L2 (159.7, 174) -> (60.3, 174)
  line L3 (60.3, 174) -> (60.3, 170)
  dimension "d1028" = 170
  dimension "d1029" = 99.4
  dimension "d1030" = 4
  constraint horizontal L0
  constraint vertical L1
  constraint horizontal L2
  constraint vertical L3
  measures "d1028" vertical distance of origin L0.start
  measures "d1029" horizontal distance of L0.start L0.end
  measures "d1030" vertical distance of L0.end L1.end
extrude "Drain slot 14''" cut sketch "草图15 (3)" along normal blind 4 bodies 10 in component "LS_RemovableGrate"
ref_plane "工作平面16" through (0, 0, 26) normal (0, 0, 1) x (1, 0, 0) in component "LS_RemovableGrate"
sketch "草图16 (3)" plane through (0, 0, 26) normal (0, 0, 1) x (1, 0, 0) in component "LS_RemovableGrate"
  line L0 (60.3, 160) -> (159.7, 160)
  line L1 (159.7, 160) -> (159.7, 164)
  line L2 (159.7, 164) -> (60.3, 164)
  line L3 (60.3, 164) -> (60.3, 160)
  dimension "d1036" = 160
  dimension "d1037" = 99.4
  dimension "d1038" = 4
  constraint horizontal L0
  constraint vertical L1
  constraint horizontal L2
  constraint vertical L3
  measures "d1036" vertical distance of origin L0.start
  measures "d1037" horizontal distance of L0.start L0.end
  measures "d1038" vertical distance of L0.end L1.end
extrude "Drain slot 15''" cut sketch "草图16 (3)" along normal blind 4 bodies 10 in component "LS_RemovableGrate"
chamfer "倒角1'''''''''" distance 0.4 angle 45 4 edges at (110, 318.7, 30) (166.7, 232, 30) (110, 145.3, 30) (53.3, 232, 30) on bodies 10 in component "LS_RemovableGrate"
ref_plane "工作平面1" through (0, 0, 10) normal (0, 0, 1) x (1, 0, 0) in component "RS_Integrated"
sketch "草图1 (11)" plane through (0, 0, 10) normal (0, 0, 1) x (1, 0, 0) in component "RS_Integrated"
  line L0 (770, 142) -> (860, 142)
  line L1 (860, 142) -> (860, 322)
  line L2 (860, 322) -> (770, 322)
  line L3 (770, 322) -> (770, 142)
  dimension "d1044" = 770
  dimension "d1045" = 142
  dimension "d1046" = 90
  dimension "d1047" = 180
  constraint horizontal L0
  constraint vertical L1
  constraint horizontal L2
  constraint vertical L3
  measures "d1044" horizontal distance of origin L0.start
  measures "d1045" vertical distance of origin L0.start
  measures "d1046" horizontal distance of L0.start L0.end
  measures "d1047" vertical distance of L0.end L1.end
extrude "R05 pan blank'''''" add sketch "草图1 (11)" along normal blind 25 separate body makes body 11 in component "RS_Integrated"
fillet "Outside corner rounds'''''" radius 3 4 edges at (770, 322, 22.5) (860, 322, 22.5) (860, 142, 22.5) (770, 142, 22.5) on bodies 11 in component "RS_Integrated"
ref_plane "工作平面2" through (0, 145, 0) normal (0, 1, 0) x (0, 0, 1) in component "RS_Integrated"
sketch "草图2 (11)" plane through (0, 145, 0) normal (0, 1, 0) x (1, 0, 0) in component "RS_Integrated"
  line L0 (857, -22.1441) -> (770, -13)
  line L1 (770, -13) -> (770, -36)
  line L2 (770, -36) -> (857, -36)
  line L3 (857, -36) -> (857, -22.1441)
  dimension "d1054" = 857
  dimension "d1055" = 22.1441
  dimension "d1056" = 770
  dimension "d1057" = 13
  dimension "d1058" = 36
  constraint vertical L1
  constraint horizontal L2
  constraint vertical L3
  measures "d1054" horizontal distance of origin L0.start
  measures "d1055" vertical distance of origin L0.start
  measures "d1056" horizontal distance of origin L0.end
  measures "d1057" vertical distance of origin L0.end
  measures "d1058" vertical distance of origin L1.end
extrude "R05 continuous slope and open edge'''''" cut sketch "草图2 (11)" along normal blind 174 bodies 11 in component "RS_Integrated"
ref_plane "工作平面3" through (0, 0, 10) normal (0, 0, 1) x (1, 0, 0) in component "RS_Integrated"
sketch "草图3 (11)" plane through (0, 0, 10) normal (0, 0, 1) x (1, 0, 0) in component "RS_Integrated"
  line L0 (857, 145) -> (845, 152)
  line L1 (845, 152) -> (833, 145)
  line L2 (833, 145) -> (857, 145)
  dimension "d1063" = 857
  dimension "d1065" = 845
  dimension "d1067" = 833
  constraint horizontal L2
  measures "d1063" horizontal distance of origin L0.start
  measures "d1065" horizontal distance of origin L0.end
  measures "d1067" horizontal distance of origin L1.end
extrude "R05 triangular flow seat 00'''''" add sketch "草图3 (11)" along normal blind 16 bodies 11 in component "RS_Integrated"
fillet "R05 soften flow seat tip'''''" radius 1 1 edges at (845, 152, 23.4414) on bodies 11 in component "RS_Integrated"
ref_plane "工作平面4" through (0, 0, 10) normal (0, 0, 1) x (1, 0, 0) in component "RS_Integrated"
sketch "草图4 (11)" plane through (0, 0, 10) normal (0, 0, 1) x (1, 0, 0) in component "RS_Integrated"
  line L0 (797, 145) -> (785, 152)
  line L1 (785, 152) -> (773, 145)
  line L2 (773, 145) -> (797, 145)
  dimension "d1074" = 797
  dimension "d1076" = 785
  dimension "d1078" = 773
  constraint horizontal L2
  measures "d1074" horizontal distance of origin L0.start
  measures "d1076" horizontal distance of origin L0.end
  measures "d1078" horizontal distance of origin L1.end
extrude "R05 triangular flow seat 01'''''" add sketch "草图4 (11)" along normal blind 16 bodies 11 in component "RS_Integrated"
fillet "R05 soften flow seat tip (1)'''''" radius 1 1 edges at (785, 152, 20.2883) on bodies 11 in component "RS_Integrated"
ref_plane "工作平面5" through (0, 0, 10) normal (0, 0, 1) x (1, 0, 0) in component "RS_Integrated"
sketch "草图5 (11)" plane through (0, 0, 10) normal (0, 0, 1) x (1, 0, 0) in component "RS_Integrated"
  line L0 (857, 319) -> (845, 312)
  line L1 (845, 312) -> (833, 319)
  line L2 (833, 319) -> (857, 319)
  dimension "d1085" = 857
  dimension "d1087" = 845
  dimension "d1089" = 833
  constraint horizontal L2
  measures "d1085" horizontal distance of origin L0.start
  measures "d1087" horizontal distance of origin L0.end
  measures "d1089" horizontal distance of origin L1.end
extrude "R05 triangular flow seat 10'''''" add sketch "草图5 (11)" along normal blind 16 bodies 11 in component "RS_Integrated"
fillet "R05 soften flow seat tip (2)'''''" radius 1 1 edges at (845, 312, 23.4414) on bodies 11 in component "RS_Integrated"
ref_plane "工作平面6" through (0, 0, 10) normal (0, 0, 1) x (1, 0, 0) in component "RS_Integrated"
sketch "草图6 (11)" plane through (0, 0, 10) normal (0, 0, 1) x (1, 0, 0) in component "RS_Integrated"
  line L0 (797, 319) -> (785, 312)
  line L1 (785, 312) -> (773, 319)
  line L2 (773, 319) -> (797, 319)
  dimension "d1096" = 797
  dimension "d1098" = 785
  dimension "d1100" = 773
  constraint horizontal L2
  measures "d1096" horizontal distance of origin L0.start
  measures "d1098" horizontal distance of origin L0.end
  measures "d1100" horizontal distance of origin L1.end
extrude "R05 triangular flow seat 11'''''" add sketch "草图6 (11)" along normal blind 16 bodies 11 in component "RS_Integrated"
fillet "R05 soften flow seat tip (3)'''''" radius 1 1 edges at (785, 312, 20.2883) on bodies 11 in component "RS_Integrated"
ref_plane "工作平面7" through (0, 0, 0) normal (0, 0, 1) x (1, 0, 0) in component "RS_Integrated"